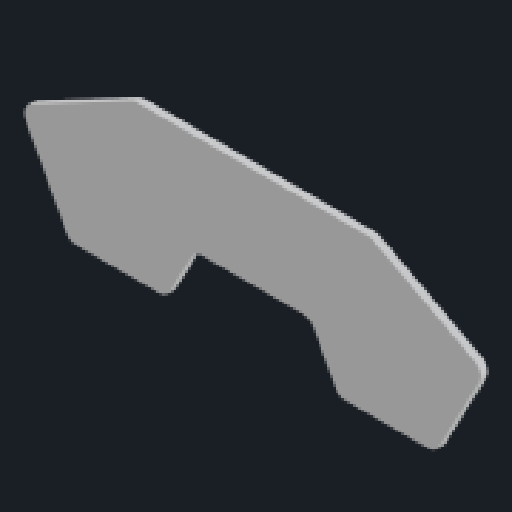
# Autodesk Inventor part: Panel
Saved by Autodesk Inventor 2023 (Build 270158000, 158)
## iProperties
Created: 2023-06-08
Part Number: Panel
Material: Generic
Document SubType Name: Modeling
Designer: valer
Density: 1 g/cm^3
Appearance: Default
Author: valer
Autodesk Inventor part; units mm, degrees
ref_plane "YZ Plane" through (0, 0, 0) normal (1, 0, 0) x (0, 1, 0)
ref_plane "XZ Plane" through (0, 0, 0) normal (0, 1, 0) x (-1, 0, 0)
ref_plane "XY Plane" through (0, 0, 0) normal (0, 0, 1) x (1, 0, 0)
sketch "Sketch2" plane through (0, 0, 0) normal (0, 0, 1) x (1, 0, 0)
  arc A0 (16.7755, -14.2265) -> (13.9693, -12.5367) centre (13.9693, -15.7117) ccw construction
  line L0 (-14.211, -12.5367) -> (13.9693, -12.5367) construction
  arc A1 (-14.211, -12.5367) -> (-17.0172, -14.2265) centre (-14.211, -15.7117) ccw construction
  line L1 (-23.1148, -25.7478) -> (-17.0172, -14.2265) construction
  arc A2 (-25.9211, -27.4376) -> (-23.1148, -25.7478) centre (-25.9211, -24.2626) ccw construction
  line L2 (-48.8874, -27.4376) -> (-25.9211, -27.4376) construction
  arc A3 (-51.6936, -25.7478) -> (-48.8874, -27.4376) centre (-48.8874, -24.2626) ccw construction
  line L3 (-63.018, -4.3507) -> (-51.6936, -25.7478) construction
  arc A4 (-61.697, -0.0593) -> (-63.018, -4.3507) centre (-60.2118, -2.8655) ccw construction
  line L4 (-33.5768, 14.8234) -> (-61.697, -0.0593) construction
  arc A5 (-32.0916, 15.1921) -> (-33.5768, 14.8234) centre (-32.0916, 12.0171) ccw construction
  line L5 (31.8499, 15.1921) -> (-32.0916, 15.1921) construction
  arc A6 (33.3351, 14.8234) -> (31.8499, 15.1921) centre (31.8499, 12.0171) ccw construction
  line L6 (61.4553, -0.0593) -> (33.3351, 14.8234) construction
  arc A7 (62.7763, -4.3507) -> (61.4553, -0.0593) centre (59.9701, -2.8655) ccw construction
  line L7 (51.4519, -25.7478) -> (62.7763, -4.3507) construction
  arc A8 (48.6457, -27.4376) -> (51.4519, -25.7478) centre (48.6457, -24.2626) ccw construction
  line L8 (25.6793, -27.4376) -> (48.6457, -27.4376) construction
  arc A9 (22.8731, -25.7478) -> (25.6793, -27.4376) centre (25.6793, -24.2626) ccw construction
  line L9 (16.7755, -14.2265) -> (22.8731, -25.7478) construction
  circle A10 centre (-67.2065, -0.7123) radius 1
  circle A11 centre (-22.8048, -29.4376) radius 1
  circle A12 centre (14.6768, -14.5367) radius 1
  circle A13 centre (66.9647, -0.7123) radius 1
  circle A14 centre (-33.3766, 17.1921) radius 1
  circle A15 centre (33.1349, 17.1921) radius 1
  circle A16 centre (51.7619, -29.4376) radius 1
  circle A17 centre (-14.9185, -14.5367) radius 1
  circle A18 centre (-52.0036, -29.4376) radius 1
  arc A19 (20.4644, -29.7478) -> (23.2707, -31.4376) centre (23.2707, -28.2626) ccw
  line L10 (51.0543, -31.4376) -> (23.2707, -31.4376)
  arc A20 (51.0543, -31.4376) -> (53.8605, -29.7478) centre (51.0543, -28.2626) ccw
  line L11 (68.1828, -2.6864) -> (53.8605, -29.7478)
  arc A21 (68.1828, -2.6864) -> (66.8618, 1.605) centre (65.3766, -1.2012) ccw
  line L12 (34.3283, 18.8234) -> (66.8618, 1.605)
  arc A22 (34.3283, 18.8234) -> (32.8431, 19.1921) centre (32.8431, 16.0171) ccw
  line L13 (-33.0848, 19.1921) -> (32.8431, 19.1921)
  arc A23 (-33.0848, 19.1921) -> (-34.57, 18.8234) centre (-33.0848, 16.0171) ccw
  line L14 (-67.1035, 1.605) -> (-34.57, 18.8234)
  arc A24 (-67.1035, 1.605) -> (-68.4245, -2.6864) centre (-65.6183, -1.2012) ccw
  line L15 (-54.1023, -29.7478) -> (-68.4245, -2.6864)
  arc A25 (-54.1023, -29.7478) -> (-51.2961, -31.4376) centre (-51.2961, -28.2626) ccw
  line L16 (-23.5124, -31.4376) -> (-51.2961, -31.4376)
  arc A26 (-23.5124, -31.4376) -> (-20.7062, -29.7478) centre (-23.5124, -28.2626) ccw
  line L17 (-14.6085, -18.2265) -> (-20.7062, -29.7478)
  arc A27 (-11.8023, -16.5367) -> (-14.6085, -18.2265) centre (-11.8023, -19.7117) ccw
  line L18 (11.5606, -16.5367) -> (-11.8023, -16.5367)
  arc A28 (14.3668, -18.2265) -> (11.5606, -16.5367) centre (11.5606, -19.7117) ccw
  line L19 (20.4644, -29.7478) -> (14.3668, -18.2265)
  point P0 (0, 0)
  constraints: 40 end point, 40 point on circle, 29 centre point
extrude "Extrusion2" add sketch "Sketch2" along normal blind 2
sketch "Sketch3" plane through (0, 0, 2) normal (0, 0, 1) x (1, 0, 0)
  arc A0 (-25.4397, -14.7587) -> (-24.4397, -13.7587) centre (-25.4397, -13.7587) ccw
  line L0 (-25.4397, -14.7587) -> (-46.3826, -14.7587)
  arc A1 (-47.3826, -13.7587) -> (-46.3826, -14.7587) centre (-46.3826, -13.7587) ccw
  line L1 (-35.9112, -14.7587) -> (-35.9112, 2.5133) construction
  line L2 (-24.4397, -6.1227) -> (-35.9112, -6.1227) construction
  arc A2 (-24.4397, 1.5133) -> (-25.4397, 2.5133) centre (-25.4397, 1.5133) ccw
  line L3 (-25.4397, 2.5133) -> (-46.3826, 2.5133)
  line L4 (-24.4397, 1.5133) -> (-24.4397, -13.7587)
  arc A3 (-46.3826, 2.5133) -> (-47.3826, 1.5133) centre (-46.3826, 1.5133) ccw
  line L5 (-47.3826, 1.5133) -> (-47.3826, -13.7587)
  line L6 (-51.2961, -31.4376) -> (-23.5124, -31.4376) projected
  line L7 (32.8431, 19.1921) -> (-33.0848, 19.1921) projected
  line L8 (-34.57, 18.8234) -> (-67.1035, 1.605) projected
  line L9 (-11.8023, -16.5367) -> (11.5606, -16.5367) projected
  line L10 (-0.1209, -16.5367) -> (-0.1209, 19.1921) construction
  arc A4 (24.198, -13.7587) -> (25.198, -14.7587) centre (25.198, -13.7587) ccw
  line L11 (25.198, -14.7587) -> (46.1408, -14.7587)
  arc A5 (46.1408, -14.7587) -> (47.1408, -13.7587) centre (46.1408, -13.7587) ccw
  arc A6 (25.198, 2.5133) -> (24.198, 1.5133) centre (25.198, 1.5133) ccw
  line L12 (25.198, 2.5133) -> (46.1408, 2.5133)
  line L13 (24.198, 1.5133) -> (24.198, -13.7587)
  arc A7 (47.1408, 1.5133) -> (46.1408, 2.5133) centre (46.1408, 1.5133) ccw
  line L14 (47.1408, 1.5133) -> (47.1408, -13.7587)
  point P0 (0, 0)
  dimension "d10" = 22.9428
  dimension "d11" = 17.272
  dimension "d12" = 1
  dimension "d13" = 16.6789
  dimension "d15" = 16.6789
  dimension "d16" = 8.89
  constraints: 22 end point, 18 symmetric about line, 16 point on circle, 8 centre point, 5 midpoint, 4 tangent, 1 equal radius, 1 perpendicular, 1 vertical, 6 other
  measures "d10" distance between parallel lines of L5 L4
  measures "d11" distance between parallel lines of L3 L0
  measures "d12" radius of A1
  measures "d13" distance between parallel lines of L6 L0
  measures "d15" distance between parallel lines of L7 L3
  measures "d16" distance from line of L8 L3.end
extrude "Extrusion3" cut sketch "Sketch3" along normal through all both and the other way through all
equation "\"d13\" = d15"
body "Solid2"
